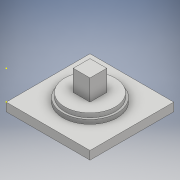
# Autodesk Inventor part: BTN_2
Saved by Autodesk Inventor 2017 (Build 210142000, 142)
## iProperties
Created: 2019-09-14
Part Number: BTN_2
Material: Generic
Document SubType Name: Modeling
Designer: Admin
Density: 1 g/cm^3
Appearance: Default
Mass: 0.140729 g
Surface Area: 2.79635 cm^2
Volume: 0.140729 cm^3
Author: Admin
Autodesk Inventor part; units mm, degrees
ref_plane "YZ Plane" through (0, 0, 0) normal (1, 0, 0) x (0, 1, 0)
ref_plane "XZ Plane" through (0, 0, 0) normal (0, 1, 0) x (-1, 0, 0)
ref_plane "XY Plane" through (0, 0, 0) normal (0, 0, 1) x (1, 0, 0)
sketch "Sketch1" plane through (0, 0, 0) normal (0, 0, 1) x (1, 0, 0)
  line L0 (0, 0) -> (10, 0)
  line L1 (10, 0) -> (10, 10)
  line L2 (10, 10) -> (0, 10)
  line L3 (0, 10) -> (0, 0)
  dimension "d0" = 10
  dimension "d1" = 10
  constraints: 8 end point, 3 perpendicular, 1 horizontal
  measures "d0" distance of L0.start L0.end
  measures "d1" distance of L0.end L1.end
extrude "Extrusion1" add sketch "Sketch1" along normal blind 1
sketch "Sketch2" plane through (0, 0, 1) normal (0, 0, 1) x (1, 0, 0)
  line L0 (10, 10) -> (0, 10) projected
  line L1 (5, 10) -> (5, 5)
  circle A0 centre (5, 5) radius 3.25
  point P0 (0, 0)
  dimension "d4" = 5
  dimension "d5" = 6.5
  constraints: 2 end point, 1 centre point, 1 coincident, 1 midpoint, 1 vertical
  measures "d4" distance of L1.start L1.end
  measures "d5" diameter of A0
extrude "Extrusion2" add sketch "Sketch2" along normal blind 0.5
sketch "Sketch3" plane through (5, 5, 1.5) normal (0, 0, 1) x (1, 0, 0)
  circle A0 centre (0, 0) radius 3
  point P0 (-5, -5)
  dimension "d8" = 6
  constraints: 1 centre point
  measures "d8" diameter of A0
extrude "Extrusion3" add sketch "Sketch3" along normal blind 0.5
sketch "Sketch4" plane through (5, 5, 2) normal (0, 0, 1) x (1, 0, 0)
  line L0 (1, 0) -> (1, 1)
  line L1 (1, 1) -> (-1, 1)
  line L2 (-1, 1) -> (-1, -1)
  line L3 (-1, -1) -> (1, -1)
  line L4 (1, -1) -> (1, 0)
  point P0 (-5, -5)
  dimension "d12" = 1
  dimension "d13" = 2
  dimension "d14" = 2
  constraints: 10 end point, 4 perpendicular, 1 point on line
  measures "d12" distance of L0.start L0.end
  measures "d13" distance of L0.end L1.end
  measures "d14" distance of L1.end L2.end
extrude "Extrusion4" add sketch "Sketch4" along normal blind 2.5
sketch "Sketch5" plane through (0, 0, 1) normal (0, 0, 1) x (1, 0, 0)
  point P0 (0, 0)
sketch "Sketch6" plane through (5, 5, 4.5) normal (0, 0, 1) x (1, 0, 0)
  point P0 (-5, -5)
body "Solid1"
